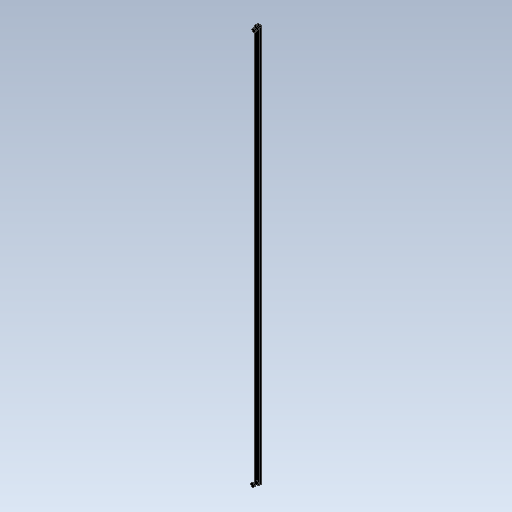
# Autodesk Inventor part: Lenkung_verbindung
Saved by Autodesk Inventor 2020.3 (Build 243373000, 373)
## iProperties
Created: 2020-02-25
Part Number: Lenkung_verbindung
Material: Generisch
Document SubType Name: Modeling
Designer: Stefan
Density: 1 g/cm^3
Appearance: Vorgabe
Mass: 346.982 g
Surface Area: 1047.9 cm^2
Volume: 346.982 cm^3
Author: Stefan
Autodesk Inventor part; units mm, degrees
ref_plane "YZ Plane" through (0, 0, 0) normal (1, 0, 0) x (0, 1, 0)
ref_plane "XZ Plane" through (0, 0, 0) normal (0, 1, 0) x (-1, 0, 0)
ref_plane "XY Plane" through (0, 0, 0) normal (0, 0, 1) x (1, 0, 0)
sketch "Skizze1" plane through (0, 0, 0) normal (0, 0, 1) x (1, 0, 0)
  line L0 (-15, 1712.029) -> (-5, 1712.029)
  line L1 (0, 1707.029) -> (0, 5)
  line L2 (-5, 0) -> (-15, 0)
  line L3 (-20, 5) -> (-20, 1707.029)
  circle A0 centre (-10, 10) radius 5.95
  circle A1 centre (-10, 1702.029) radius 5.95
  arc A2 (-15, 1712.029) -> (-20, 1707.029) centre (-15, 1707.029) ccw
  arc A3 (0, 1707.029) -> (-5, 1712.029) centre (-5, 1707.029) ccw
  arc A4 (-20, 5) -> (-15, 0) centre (-15, 5) ccw
  arc A5 (-5, 0) -> (0, 5) centre (-5, 5) ccw
  point P0 (0, 0)
  point P1 (-20, 1712.029)
  point P2 (0, 1712.029)
  dimension "d0" = 20
  dimension "d2" = 11.9
  dimension "d3" = 10
  dimension "d4" = 10
  dimension "d5" = 11.9
  dimension "d6" = 10
  dimension "d7" = 1692.029
  dimension "d8" = 10
  dimension "d9" = 5
  constraints: 8 end point, 8 point on circle, 8 tangent, 6 centre point, 6 point on line, 3 equal radius, 2 parallel, 1 horizontal, 1 perpendicular
  measures "d0" distance of point (-20, 1712.029) point (0, 1712.029)
  measures "d2" diameter of A0
  measures "d3" distance from line of A0.centre L1
  measures "d4" distance from line of L2 A0.centre
  measures "d5" diameter of A1
  measures "d6" distance from line of L1 A1.centre
  measures "d7" distance of A0.centre A1.centre
  measures "d8" distance from line of L0 A1.centre
  measures "d9" radius of A2
extrude "Extrusion1" add sketch "Skizze1" against normal blind 10 contours L0 A3 L1 A5 L2 A4 L3 A2 | A0 | A1
extrude "Extrusion2" add sketch "Skizze1" along normal blind 10 contours A1
sketch "Skizze2" plane through (-10, 1702.029, 10) normal (0, 0, 1) x (1, 0, 0)
  circle A0 centre (0, 0) radius 8
  point P0 (10, -1702.029)
  dimension "d14" = 16
  constraints: 1 centre point
  measures "d14" diameter of A0
extrude "Extrusion3" add sketch "Skizze2" along normal blind 5
extrude "Extrusion4" add sketch "Skizze1" along normal blind 15 contours A0
sketch "Skizze3" plane through (-10, 10, 15) normal (0, 0, 1) x (1, 0, 0)
  circle A0 centre (0, 0) radius 8
  point P0 (10, -10)
  dimension "d19" = 16
  constraints: 1 centre point
  measures "d19" diameter of A0
extrude "Extrusion5" add sketch "Skizze3" along normal blind 5
